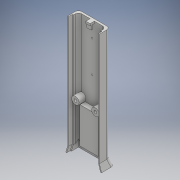
# Autodesk Inventor part: Case bengala
Saved by Autodesk Inventor 2018 (Build 220112000, 112)
## iProperties
Created: 2017-10-19
Part Number: Case bengala
Material: Genérico
Document SubType Name: Modeling
Designer: mirre
Density: 1 g/cm^3
Appearance: Padrão
Author: mirre
Autodesk Inventor part; units mm, degrees
ref_plane "YZ Plane" through (0, 0, 0) normal (1, 0, 0) x (0, 1, 0)
ref_plane "XZ Plane" through (0, 0, 0) normal (0, 1, 0) x (-1, 0, 0)
sketch "Esboço1" plane through (0, 0, 0) normal (0, 0, 1) x (1, 0, 0)
  line L0 (0, 0) -> (52, 0)
  line L1 (52, 0) -> (52, 37)
  line L2 (52, 37) -> (0, 37)
  line L3 (0, 37) -> (0, 0)
  dimension "d0" = 37
  dimension "d1" = 52
  constraints: 8 end point, 3 perpendicular, 1 horizontal
  measures "d0" distance of L2.end L0.start
  measures "d1" distance of L0.start L0.end
extrude "Extrusão1" add sketch "Esboço1" along normal blind 5
sketch "Esboço2" plane through (0, 0, 5) normal (0, 0, 1) x (1, 0, 0)
  circle A0 centre (12.95, 24) radius 8.05
  circle A1 centre (39.05, 24) radius 8.05
  line L0 (52, 37) -> (0, 37) projected
  line L1 (0, 37) -> (0, 0) projected
  dimension "d4" = 16.1
  dimension "d5" = 16.1
  dimension "d6" = 26.1
  dimension "d8" = 13
  dimension "d9" = 13
  dimension "d13" = 12.95
  constraints: 2 centre point
  measures "d4" diameter of A1
  measures "d5" diameter of A0
  measures "d6" distance of A1.centre A0.centre
  measures "d8" distance from line of L0 A0.centre
  measures "d9" distance from line of L0 A1.centre
  measures "d13" distance from line of L1 A0.centre
extrude "Extrusão2" cut sketch "Esboço2" against normal through all
sketch "Esboço3" plane through (0, 0, 5) normal (0, 0, 1) x (1, 0, 0)
  line L0 (20.5, 34) -> (20.5, 28.5)
  line L1 (20.5, 28.5) -> (31.5, 28.5)
  line L2 (31.5, 28.5) -> (31.5, 34)
  line L3 (31.5, 34) -> (20.5, 34)
  line L4 (52, 37) -> (0, 37) projected
  line L5 (52, 0) -> (52, 37) projected
  line L6 (20.5, 14) -> (20.5, 19)
  line L7 (20.5, 19) -> (31.5, 19)
  line L8 (31.5, 19) -> (31.5, 14)
  line L9 (31.5, 14) -> (20.5, 14)
  line L10 (0, 0) -> (52, 0) projected
  dimension "d16" = 3
  dimension "d17" = 5.5
  dimension "d19" = 20.5
  dimension "d39" = 5
  dimension "d40" = 14
  dimension "d234" = 11
  dimension "d235" = 11
  constraints: 16 end point, 6 perpendicular, 2 collinear, 1 horizontal, 1 vertical
  measures "d16" distance between parallel lines of L4 L3
  measures "d17" distance of L1.end L2.end
  measures "d19" distance between parallel lines of L5 L2
  measures "d39" distance of L7.end L8.end
  measures "d40" distance between parallel lines of L10 L9
  measures "d234" distance of L0.end L1.end
  measures "d235" distance of L6.end L7.end
extrude "Extrusão3" cut sketch "Esboço3" against normal blind 4
sketch "Esboço5" plane through (0, 0, 0) normal (0, 0, -1) x (-1, 0, 0)
  circle A0 centre (-39.05, 24) radius 9.05
  circle A1 centre (-12.95, 24) radius 9.05
  circle A2 centre (-39.05, 24) radius 8.05 projected
  circle A3 centre (-12.95, 24) radius 8.05 projected
  point P0 (0, 0)
  dimension "d30" = 1
  dimension "d31" = 1
  dimension "d32" = 16.1
  dimension "d34" = 16.1
  constraints: 2 centre point, 2 concentric
  measures "d30" radial gap between concentric circles of A0 A2
  measures "d31" radial gap between concentric circles of A1 A3
  measures "d32" diameter of A3
  measures "d34" diameter of A2
extrude "Extrusão5" add sketch "Esboço5" along normal blind 7
sketch "Esboço6" plane through (0, 0, 5) normal (0, 0, 1) x (1, 0, 0)
  line L0 (52, 37) -> (0, 37) projected
  line L1 (0, 0) -> (52, 0) projected
  line L2 (0, 37) -> (0, 0)
  line L3 (0, 0) -> (52, 0)
  line L4 (52, 0) -> (52, 37) projected
  line L5 (52, 0) -> (52, 37)
  line L6 (52, 37) -> (0, 37)
  line L7 (3, 34) -> (3, 3)
  line L8 (3, 3) -> (49, 3)
  line L9 (49, 3) -> (49, 34)
  line L10 (49, 34) -> (3, 34)
  dimension "d43" = 3
  dimension "d44" = 3
  dimension "d45" = 3
  dimension "d46" = 3
  constraints: 16 end point, 6 perpendicular, 1 collinear, 1 vertical
  measures "d43" distance between parallel lines of L0 L10
  measures "d44" distance between parallel lines of L1 L8
  measures "d45" distance between parallel lines of L2 L7
  measures "d46" distance between parallel lines of L4 L9
extrude "Extrusão6" add sketch "Esboço6" along normal blind 5
ref_plane "Plano de trabalho1" through (0, 0, 20) normal (0, 0, 1) x (1, 0, 0)
sketch "Esboço60" plane through (0, 0, 20) normal (0, 0, 1) x (1, 0, 0)
  line L0 (3, 18.5) -> (3, 34)
  line L1 (3, 34) -> (49, 34) projected
  line L2 (3, 34) -> (49, 34)
  line L3 (49, 34) -> (49, 18.5)
  line L4 (49, 18.5) -> (46, 18.5)
  line L5 (46, 18.5) -> (46, 31)
  line L6 (46, 31) -> (6, 31)
  line L7 (6, 31) -> (6, 18.5)
  line L8 (6, 18.5) -> (3, 18.5)
  point P0 (0, 0)
  dimension "d400" = 3
  dimension "d401" = 12.5
  dimension "d403" = 3
  dimension "d404" = 15.5
  constraints: 16 end point, 7 perpendicular, 1 point on line
  measures "d400" distance of L3.end L4.end
  measures "d401" distance of L4.end L5.end
  measures "d403" distance between parallel lines of L7 L0
  measures "d404" distance of L0.start L0.end
sketch "Esboço59" plane through (0, 0, 10) normal (0, 0, 1) x (1, 0, 0)
  line L0 (52, 37) -> (0, 37) projected
  line L1 (0, 37) -> (0, 18.5)
  line L2 (3, 18.5) -> (3, 34)
  line L3 (49, 34) -> (49, 18.5)
  line L4 (52, 18.5) -> (52, 37)
  line L5 (52, 37) -> (0, 37)
  line L6 (0, 18.5) -> (3, 18.5)
  line L7 (49, 18.5) -> (52, 18.5)
  line L8 (3, 34) -> (49, 34)
  line L9 (0, 37) -> (0, 0) projected
  dimension "d395" = 3
  dimension "d396" = 18.5
  dimension "d397" = 3
  dimension "d398" = 18.5
  dimension "d399" = 3
  constraints: 16 end point, 2 perpendicular, 2 vertical, 1 collinear, 1 parallel
  measures "d395" distance between parallel lines of L4 L3
  measures "d396" distance of L0.end L1.end
  measures "d397" distance of L1.end L2.start
  measures "d398" distance of L4.start L4.end
  measures "d399" distance between parallel lines of L0 L8
loft "Transição3" add profiles "Esboço60", "Esboço59"
sketch "Esboço61" plane through (3, 34, 20) normal (0, 0, 1) x (1, 0, 0)
  line L0 (0, 0) -> (46, 0) projected
  line L1 (0, -15.5) -> (3, -15.5) projected
  line L2 (0, 0) -> (0, -15.5)
  line L3 (3, -15.5) -> (3, -3) projected
  line L4 (0, -15.5) -> (3, -15.5)
  line L5 (3, -15.5) -> (3, -3)
  line L6 (3, -3) -> (43, -3) projected
  line L7 (3, -3) -> (43, -3)
  line L8 (43, -15.5) -> (46, -15.5) projected
  line L9 (43, -3) -> (43, -15.5)
  line L10 (43, -15.5) -> (46, -15.5)
  line L11 (46, -31) -> (46, 0) projected
  line L12 (46, -15.5) -> (46, 0)
  line L13 (46, 0) -> (0, 0)
  point P0 (-3, -34)
  constraints: 16 end point, 5 perpendicular, 3 collinear
extrude "Extrusão34" add sketch "Esboço61" along normal blind 163.1
sketch "Esboço64" plane through (3, 34, 183.1) normal (0, 0, 1) x (1, 0, 0)
  line L0 (3, -15.5) -> (0, -15.5) projected
  line L1 (3, -15.5) -> (3, -10.5)
  line L2 (3, -15.5) -> (3, -3) projected
  line L3 (1.5, -10.5) -> (3, -10.5)
  line L4 (1.5, -15.5) -> (3, -15.5)
  line L5 (43, -15.5) -> (43, -10.5)
  line L6 (43, -3) -> (43, -15.5) projected
  line L7 (43, -15.5) -> (46, -15.5) projected
  line L8 (44.5, -15.5) -> (43, -15.5)
  line L9 (43, -10.5) -> (44.5, -10.5)
  line L10 (1.5, -10.5) -> (1.5, -15.5)
  line L11 (44.5, -15.5) -> (44.5, -10.5)
  dimension "d420" = 5
  dimension "d424" = 1.5
  dimension "d425" = 5
  dimension "d507" = 1.5
  constraints: 16 end point, 3 perpendicular, 2 point on line, 1 collinear, 1 vertical
  measures "d420" distance of L0.start L1.end
  measures "d424" distance of L3.start L1.end
  measures "d425" distance between parallel lines of L9 L8
  measures "d507" distance of L5.end L9.end
extrude "Extrusão35" cut sketch "Esboço64" against normal blind 163.1
sketch "Esboço71" plane through (0, 0, 0) normal (-1, 0, 0) x (0, 0, 1)
  line L0 (0, 0) -> (10, 0) projected
  line L1 (10, 0) -> (-34.6631, 0)
  line L2 (-34.6631, 0) -> (-34.6631, 49.4717)
  line L3 (-34.6631, 49.4717) -> (10, 49.4717)
  line L4 (10, 49.4717) -> (10, 0)
  constraints: 8 end point, 2 parallel, 1 horizontal, 1 perpendicular
extrude "Extrusão38" cut sketch "Esboço71" against normal through all
sketch "Esboço78" plane through (3, 18.5, 20) normal (0, -1, 0) x (1, 0, 0)
  line L0 (3, 0) -> (3, 163.1) projected
  line L1 (3, 0) -> (1.5, 0)
  line L2 (46, 0) -> (0, 0) projected
  line L3 (1.5, 0) -> (-1.5, -10)
  line L4 (-1.5, -10) -> (0, -10)
  line L5 (3, 0) -> (0, -10) projected
  line L6 (0, -10) -> (3, 0)
  line L7 (3, 0) -> (43, 0) projected
  line L8 (43, 0) -> (44.5, 0)
  line L9 (44.5, 0) -> (47.5, -10)
  line L10 (47.5, -10) -> (46, -10)
  line L11 (43, 0) -> (46, -10)
  dimension "d461" = 1.5
  dimension "d462" = 1.5
  dimension "d463" = 1.5
  dimension "d464" = 1.5
  constraints: 16 end point, 2 point on line, 1 collinear, 1 horizontal
  measures "d461" distance of L0.start L1.end
  measures "d462" distance of L3.end L4.end
  measures "d463" distance of L7.end L8.end
  measures "d464" distance of L9.end L10.end
extrude "Extrusão42" cut sketch "Esboço78" against normal blind 5
sketch "Esboço81" plane through (3, 34, 183.1) normal (0, 0, 1) x (1, 0, 0)
  line L0 (3, -3) -> (43, -3) projected
  line L1 (19.9, -3) -> (26.1, -3)
  line L2 (26.1, -3) -> (26.1, -9.1)
  line L3 (26.1, -9.1) -> (19.9, -9.1)
  line L4 (19.9, -9.1) -> (19.9, -3)
  line L5 (0, 0) -> (0, -15.5) projected
  dimension "d472" = 19.9
  dimension "d473" = 6.2
  dimension "d474" = 6.1
  constraints: 8 end point, 2 parallel, 1 horizontal, 1 perpendicular, 1 point on line
  measures "d472" distance between parallel lines of L5 L4
  measures "d473" distance of L2.end L3.end
  measures "d474" distance between parallel lines of L0 L3
extrude "Extrusão44" add sketch "Esboço81" against normal blind 3
sketch "Esboço82" plane through (3, 34, 20) normal (0, 1, 0) x (1, 0, 0)
  circle A0 centre (23, -140.1) radius 1
  circle A1 centre (23, -94.1) radius 1
  line L0 (0, 0) -> (0, -163.1) projected
  line L1 (46, -163.1) -> (0, -163.1) projected
  dimension "d477" = 23
  dimension "d478" = 23
  dimension "d479" = 23
  dimension "d480" = 46
  dimension "d483" = 2
  dimension "d484" = 2
  constraints: 2 centre point
  measures "d477" distance from line of A0.centre L0
  measures "d478" distance from line of L0 A1.centre
  measures "d479" distance from line of L1 A0.centre
  measures "d480" distance of A0.centre A1.centre
  measures "d483" diameter of A1
  measures "d484" diameter of A0
extrude "Extrusão45" cut sketch "Esboço82" against normal blind 3
fillet "Arredondamento6" radius 5 6 edges at (6, 31, 101.55) (49, 34, 101.55) (1.5, 35.5, 15) (50.5, 35.5, 15) (46, 31, 101.55) (3, 34, 101.55)
sketch "Esboço84" plane through (8, 34, 183.1) normal (0, 1, 0) x (1, 0, 0)
  circle A0 centre (3.5, 103.6) radius 3.45
  circle A1 centre (32.5, 103.6) radius 3.45
  line L0 (36, 0) -> (0, 0) projected
  line L1 (41, 0) -> (41, 163.1) projected
  line L2 (-5, 163.1) -> (-5, 0) projected
  point P0 (-8, 183.1)
  point P1 (-2, 0)
  point P2 (38, 0)
  dimension "d488" = 103.6
  dimension "d491" = 103.6
  dimension "d492" = 6.9
  dimension "d493" = 6.9
  dimension "d496" = 8.5
  dimension "d497" = 8.5
  constraints: 2 centre point
  measures "d488" distance from line of L0 A0.centre
  measures "d491" distance from line of L0 A1.centre
  measures "d492" diameter of A0
  measures "d493" diameter of A1
  measures "d496" distance from line of L1 A1.centre
  measures "d497" distance from line of A0.centre L2
extrude "Extrusão46" cut sketch "Esboço84" against normal through all
sketch "Esboço85" plane through (3, 34, 180.1) normal (0, 0, -1) x (-1, 0, 0)
  line L0 (-26.1, -5.65) -> (-19.9, -5.65)
  line L1 (-19.9, -5.65) -> (-19.9, -7.65)
  line L2 (-19.9, -7.65) -> (-26.1, -7.65)
  line L3 (-26.1, -7.65) -> (-26.1, -5.65)
  line L4 (-19.9, -9.1) -> (-19.9, -3) projected
  line L5 (-26.1, -3) -> (-26.1, -9.1) projected
  line L6 (-26.1, -9.1) -> (-19.9, -9.1) projected
  point P0 (3, -34)
  dimension "d499" = 1.45
  dimension "d500" = 2
  constraints: 8 end point, 2 collinear, 2 parallel, 1 horizontal, 1 perpendicular
  measures "d499" distance between parallel lines of L6 L2
  measures "d500" distance between parallel lines of L2 L0
extrude "Extrusão47" add sketch "Esboço85" along normal blind 6 contours L0 L1 L2 L3
sketch "Esboço88" plane through (22.9, 31, 180.1) normal (0, -1, 0) x (1, 0, 0)
  arc A0 (-11.9, -104.0136) -> (-11.9, -97.1864) centre (-11.4, -100.6) ccw projected
  circle A1 centre (-11.4, -100.6) radius 3.45
  circle A2 centre (-11.4, -100.6) radius 5.45
  arc A3 (18.1, -97.1864) -> (18.1, -104.0136) centre (17.6, -100.6) ccw projected
  circle A4 centre (17.6, -100.6) radius 3.45
  circle A5 centre (17.6, -100.6) radius 5.45
  point P0 (-22.9, -180.1)
  dimension "d508" = 2
  dimension "d510" = 2
  constraints: 4 centre point, 4 coincident
  measures "d508" radial gap between concentric circles of A2 A0
  measures "d510" radial gap between concentric circles of A5 A3
extrude "Extrusão49" add sketch "Esboço88" along normal blind 10
sketch "Esboço89" plane through (40.5, 21, 79.5) normal (0, -1, 0) x (1, 0, 0)
  circle A0 centre (0, 0) radius 2
  circle A1 centre (0, 0) radius 3.45 projected
  circle A2 centre (-29, 0) radius 2
  circle A3 centre (-29, 0) radius 3.45
  circle A4 centre (0, 0) radius 3.45
  point P0 (-40.5, -79.5)
  dimension "d513" = 4
  dimension "d514" = 4
  constraints: 4 centre point, 3 coincident, 2 concentric
  measures "d513" diameter of A0
  measures "d514" diameter of A2
extrude "Extrusão50" add sketch "Esboço89" against normal blind 5
sketch "Esboço90" plane through (22.9, 31, 180.1) normal (0, -1, 0) x (1, 0, 0)
  line L0 (19.1, -157.1) -> (-7.3, -157.1)
  line L1 (-7.3, -157.1) -> (-7.3, -105.1)
  line L2 (-7.3, -105.1) -> (19.1, -105.1)
  line L3 (19.1, -105.1) -> (19.1, -157.1)
  line L4 (-11.9, -160.1) -> (18.1, -160.1) projected
  line L5 (26.1, -160.1) -> (26.1, 3) projected
  dimension "d517" = 3
  dimension "d518" = 7
  dimension "d519" = 26.4
  dimension "d520" = 52
  constraints: 8 end point, 2 parallel, 1 horizontal, 1 perpendicular
  measures "d517" distance between parallel lines of L4 L0
  measures "d518" distance between parallel lines of L5 L3
  measures "d519" distance between parallel lines of L3 L1
  measures "d520" distance between parallel lines of L2 L0
extrude "Extrusão51" add sketch "Esboço90" along normal blind 7.4
